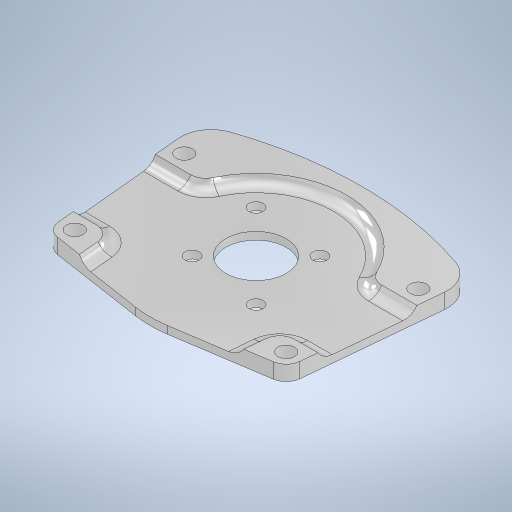
# Autodesk Inventor part: Top Plate
Saved by Autodesk Inventor 2023.2 (Build 272271000, 271)
## iProperties
Created: 2022-12-28
Part Number: Top Plate
Material: Aluminum 6061
Document SubType Name: Modeling
Designer: Nathan Cai
Mass: 6.57116 g
Surface Area: 52.7177 cm^2
Volume: 5.81518 cm^3
Density: 2.7 g/cm^3
Appearance: Aluminum - Polished
Author: Nathan Cai
Autodesk Inventor part; units mm, degrees
ref_plane "YZ Plane" through (0, 0, 0) normal (1, 0, 0) x (0, 1, 0)
ref_plane "XZ Plane" through (0, 0, 0) normal (0, 1, 0) x (-1, 0, 0)
ref_plane "XY Plane" through (0, 0, 0) normal (0, 0, 1) x (1, 0, 0)
sketch "Sketch1" plane through (0, 0, 0) normal (0, 1, 0) x (-1, 0, 0)
  circle A0 centre (0, 0) radius 73.025
  line L0 (0, 0) -> (0, -73.025) construction
  line L1 (0, 0) -> (-12.6807, -71.9156)
  line L2 (0, 0) -> (12.6807, -71.9156)
  line L3 (0, 0) -> (72.3143, -10.1631)
  line L4 (0, 0) -> (64.4772, -34.2832)
  line L5 (0, 0) -> (32.0121, 65.6344)
  line L6 (0, 0) -> (52.5298, 50.7274)
  line L7 (0, 0) -> (-52.5298, 50.7274)
  line L8 (0, 0) -> (-32.0121, 65.6344)
  line L9 (0, 0) -> (-64.4772, -34.2832)
  line L10 (0, 0) -> (-72.3143, -10.1631)
  circle A1 centre (0, 0) radius 69.85
  arc A2 (4.7597, -69.6876) -> (-4.7597, -69.6876) centre (0, -69.85) ccw
  arc A3 (67.7477, -17.0079) -> (64.806, -26.0614) centre (66.4313, -21.5848) ccw
  arc A4 (37.1107, 59.1762) -> (44.8121, 53.5808) centre (41.0568, 56.5098) ccw
  arc A5 (-44.8121, 53.5808) -> (-37.1107, 59.1762) centre (-41.0568, 56.5098) ccw
  arc A6 (-64.806, -26.0614) -> (-67.7477, -17.0079) centre (-66.4313, -21.5848) ccw
  point P0 (61.6739, -32.7926)
  point P1 (69.1702, -9.7212)
  point P2 (50.2459, 48.5219)
  point P3 (30.6202, 62.7808)
  point P4 (-30.6202, 62.7808)
  point P5 (-50.2459, 48.5219)
  point P6 (-69.1702, -9.7212)
  point P7 (-61.6739, -32.7926)
  point P8 (-12.1293, -68.7888)
  point P9 (12.1293, -68.7888)
  point P10 (64.806, -26.0614)
  point P11 (67.7477, -17.0079)
  point P12 (44.8121, 53.5808)
  point P13 (37.1107, 59.1762)
  point P14 (-37.1107, 59.1762)
  point P15 (-67.7477, -17.0079)
  dimension "d0" = 146.05
  dimension "d1" = 10
  dimension "d4" = 360
  dimension "d6" = 3.175
  dimension "d10" = 9.525
  dimension "d13" = 360
  constraints: 22 end point, 15 point on circle, 7 centre point, 4 coincident, 1 point on line, 1 symmetric about line, 1 vertical, 45 other
  measures "d0" diameter of A0
  measures "d1" angle of L0 L1
  measures "d6" radial gap between concentric circles of A0 A1
  measures "d10" diameter of A2
extrude "Extrusion1" add sketch "Sketch1" along normal blind 1.5875 contours A0 L3 A1 L6 | L5 A1 L8 A0 | A1 L3 L6 | L6 L5 A1 A4 | A0 L2 A1 L4 | A1 A3 L4 L3 | L5 L8 A1 | L2 A1 A2 L1 | L4 A1 L2 | L10 A1 L7 | L7 A1 A5 L8 | L1 A1 L9 | L9 A1 A6 L10 | A0 L1 A1 L2 | L7 A1 L10 A0 | L1 A0 L9 A1 | A2 A1
fillet "Fillet1" radius 1.5875 24 edges at (30.6202, 0.7937, 62.7808) (32.0121, 0.7937, 65.6344) (-30.6202, 0.7937, 62.7808) (-32.0121, 0.7937, 65.6344) (-52.5298, 0.7937, 50.7274) (-50.2459, 0.7937, 48.5219) (52.5298, 0.7937, 50.7274) (50.2459, 0.7937, 48.5219) (64.4772, 0.7937, -34.2832) (61.6739, 0.7937, -32.7926) (72.3143, 0.7937, -10.1631) (69.1702, 0.7937, -9.7212) (-72.3143, 0.7937, -10.1631) (-69.1702, 0.7937, -9.7212) (-64.4772, 0.7937, -34.2832) (-61.6739, 0.7937, -32.7926) (37.1107, 0.7937, 59.1762) (44.8121, 0.7937, 53.5808) (-44.8121, 0.7937, 53.5808) (-37.1107, 0.7937, 59.1762) (-64.806, 0.7937, -26.0614) (-67.7477, 0.7937, -17.0079) (67.7477, 0.7937, -17.0079) (64.806, 0.7937, -26.0614)
sketch "Sketch5" plane through (0, 1.5875, 0) normal (0, 1, 0) x (1, 0, 0)
  line L0 (0, 0) -> (0, 65.0875) construction
  circle A0 centre (0, 50.8) radius 22.225
  arc A1 (63.6995, 35.7075) -> (-63.6995, 35.7075) centre (0, 0) ccw projected
  circle A2 centre (0, 50.8) radius 12.5 construction
  circle A3 centre (-24.6062, 60.325) radius 1.7526
  circle A4 centre (-24.6062, 60.325) radius 3.175 construction
  circle A5 centre (-22.225, 34.925) radius 3.175
  circle A6 centre (-22.225, 34.925) radius 1.7526
  circle A7 centre (24.6062, 60.325) radius 1.7526
  circle A8 centre (24.6062, 60.325) radius 3.175
  circle A9 centre (22.225, 34.925) radius 3.175
  circle A10 centre (22.225, 34.925) radius 1.7526
  arc A11 (-62.3874, 31.414) -> (-64.248, 27.4085) centre (0, 0) ccw projected
  arc A12 (63.6995, 35.7075) -> (-63.6995, 35.7075) centre (0, 0) ccw projected
  line L1 (-28.4451, 67.2572) -> (-25.3861, 34.6286)
  line L2 (-22.7046, 31.7864) -> (-3.3572, 28.83)
  line L3 (28.4451, 67.2572) -> (25.3861, 34.6286)
  line L4 (22.7046, 31.7864) -> (3.3572, 28.83)
  circle A13 centre (0, 50.8) radius 6.35
  circle A14 centre (0, 0) radius 73.025
  line L5 (0, 50.8) -> (-8.8388, 59.6388) construction
  circle A15 centre (0, 50.8) radius 9.5 construction
  line L6 (0, 50.8) -> (6.7175, 57.5175) construction
  circle A16 centre (-8.8388, 59.6388) radius 1.5
  circle A17 centre (6.7175, 57.5175) radius 1.5
  circle A18 centre (8.8388, 41.9612) radius 1.5
  circle A19 centre (-6.7175, 44.0825) radius 1.5
  point P0 (-63.6995, 35.7075)
  dimension "d39" = 25
  dimension "d40" = 44.45
  dimension "d78" = 19
  dimension "d41" = 3.5052
  dimension "d42" = 6.35
  dimension "d43" = 9.525
  dimension "d44" = 24.6062
  dimension "d45" = 6.35
  dimension "d46" = 3.5052
  dimension "d47" = 15.875
  dimension "d48" = 22.225
  dimension "d68" = 12.7
  dimension "d77" = 315
  dimension "d79" = 3
  dimension "d80" = 3
  dimension "d83" = 360
  constraints: 14 end point, 13 centre point, 10 coincident, 8 symmetric about line, 3 point on circle, 3 tangent, 1 perpendicular, 1 point on line, 1 vertical, 27 other
  measures "d41" diameter of A3
  measures "d42" diameter of A4
  measures "d43" vertical distance of point (0, 50.8) A3.centre
  measures "d44" horizontal distance of point (0, 50.8) A3.centre
  measures "d45" diameter of A5
  measures "d46" diameter of A6
  measures "d47" vertical distance of point (0, 50.8) A6.centre
  measures "d48" horizontal distance of point (0, 50.8) A6.centre
  measures "d68" diameter of A13
  measures "d79" diameter of A16
  measures "d80" diameter of A17
extrude "Extrusion3" cut sketch "Sketch5" against normal blind 25.4 contours A0 L4 A9 L3 A1 A14 L1 A5 L2 | A3 | A6 | A7 | A10 | A13 | A16 | A17 | A18 | A19
fillet "Fillet4" radius 6.35 2 edges at (-28.4451, 0.7937, -67.2572) (28.4451, 0.7937, -67.2572)
sketch "Sketch7" plane through (0, 1.5875, 0) normal (0, 1, 0) x (1, 0, 0)
  arc A0 (27.9955, 62.4615) -> (23.7373, 69.0593) centre (21.6732, 63.0542) ccw projected
  arc A1 (23.7373, 69.0593) -> (-23.7373, 69.0593) centre (0, 0) ccw projected
  arc A2 (-23.7373, 69.0593) -> (-27.9955, 62.4615) centre (-21.6732, 63.0542) ccw projected
  line L0 (-27.9955, 62.4615) -> (-25.3861, 34.6286) projected
  arc A3 (-25.3861, 34.6286) -> (-22.7046, 31.7864) centre (-22.225, 34.925) ccw projected
  line L1 (-22.7046, 31.7864) -> (-3.3572, 28.83) projected
  arc A4 (-3.3572, 28.83) -> (3.3572, 28.83) centre (0, 50.8) ccw projected
  line L2 (3.3572, 28.83) -> (22.7046, 31.7864) projected
  arc A5 (22.7046, 31.7864) -> (25.3861, 34.6286) centre (22.225, 34.925) ccw projected
  line L3 (25.3861, 34.6286) -> (27.9955, 62.4615) projected
  circle A6 centre (22.225, 34.925) radius 1.7526 projected
  circle A7 centre (-22.225, 34.925) radius 1.7526 projected
  circle A8 centre (0, 50.8) radius 6.35 projected
  circle A9 centre (24.6062, 60.325) radius 1.7526 projected
  circle A10 centre (-24.6062, 60.325) radius 1.7526 projected
  circle A11 centre (0, 50.8) radius 19.05
  line L4 (-18.9668, 49.0219) -> (-17.2732, 30.9565)
  line L5 (-3.3572, 28.83) -> (-22.7046, 31.7864) projected
  line L6 (-27.9955, 62.4615) -> (-25.3861, 34.6286) projected
  arc A12 (23.7373, 69.0593) -> (-23.7373, 69.0593) centre (0, 0) ccw projected
  line L7 (0, 73.025) -> (0, 28.575) construction
  line L8 (18.9668, 49.0219) -> (17.2732, 30.9565)
  circle A13 centre (-24.6062, 60.325) radius 3.175 construction
  line L9 (-25.3861, 34.6286) -> (-27.9955, 62.4615) projected
  circle A14 centre (-22.225, 34.925) radius 1.7526 projected
  arc A15 (-25.3861, 34.6286) -> (-22.7046, 31.7864) centre (-22.225, 34.925) ccw projected
  circle A16 centre (-22.225, 34.925) radius 3.175 construction
  line L10 (27.4975, 63.5) -> (-27.4975, 63.5) construction
  line L11 (-27.4975, 63.5) -> (-27.4975, 57.15) construction
  line L12 (-27.4975, 57.15) -> (27.4975, 57.15)
  line L13 (27.4975, 57.15) -> (27.4975, 63.5) construction
  line L14 (27.4975, 63.5) -> (-27.4975, 57.15) construction
  line L15 (-27.4975, 63.5) -> (27.4975, 57.15) construction
  line L16 (25.7116, 31.75) -> (-25.7116, 31.75) construction
  line L17 (-25.7116, 31.75) -> (-25.7116, 38.1) construction
  line L18 (25.7116, 38.1) -> (25.7116, 31.75) construction
  line L19 (25.7116, 31.75) -> (-25.7116, 38.1) construction
  line L20 (-25.7116, 31.75) -> (25.7116, 38.1) construction
  line L21 (-25.7116, 38.1) -> (25.7116, 38.1)
  line L22 (-25.7116, 38.1) -> (-17.2732, 38.1)
  line L23 (-17.2732, 38.1) -> (-17.2732, 30.9565)
  line L24 (-17.2732, 30.9565) -> (-25.7116, 30.9565)
  line L25 (-25.7116, 30.9565) -> (-25.7116, 38.1)
  point P0 (0, 60.325)
  point P1 (0, 34.925)
  point P2 (-17.9429, 38.1)
  point P3 (-17.9605, 57.15)
  point P4 (17.9605, 57.15)
  point P5 (27.4975, 57.15)
  point P6 (17.9429, 38.1)
  dimension "d70" = 38.1
  constraints: 38 end point, 6 horizontal, 6 parallel, 5 point on line, 4 midpoint, 3 coincident, 3 perpendicular, 3 point on circle, 3 tangent, 2 symmetric about line, 1 centre point, 7 other
extrude "Extrusion4" add sketch "Sketch7" along normal blind 1.5875 contours L3 L12 A11 L0 A2 A1 A0 | L3 A5 L2 L8 L21 | L21 L4 L1 A3 L0
fillet "Fillet6" radius 3.175 4 edges at (-17.9429, 2.3812, -38.1) (-17.9605, 2.3812, -57.15) (17.9605, 2.3812, -57.15) (17.9429, 2.3812, -38.1)
fillet "Fillet7" radius 3.175 11 edges at (-18.6965, 1.5875, -37.2725) (-23.2729, 1.5875, -38.1) (-17.4731, 1.5875, -33.0889) (0, 1.5875, -69.85) (18.3834, 1.5875, -57.6416) (23.789, 1.5875, -57.15) (-23.789, 1.5875, -57.15) (-18.3834, 1.5875, -57.6416) (18.6965, 1.5875, -37.2725) (17.4731, 1.5875, -33.0889) (23.2729, 1.5875, -38.1)
equation "\"d45\" = d42"
equation "\"d46\" = d41"
body "Solid1"
